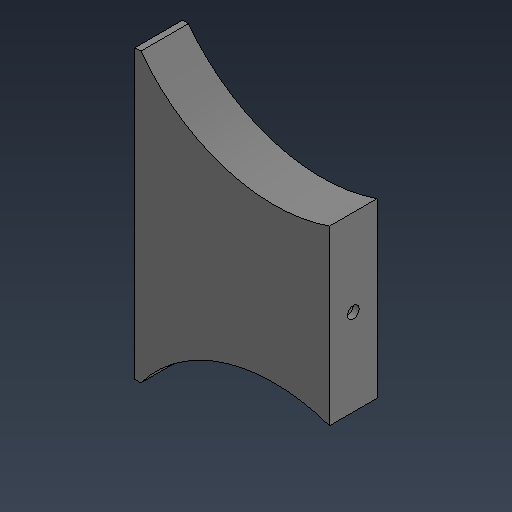
# Autodesk Inventor part: GearboxBearingHolderCover
Saved by Autodesk Inventor 2026.2 (Build 302298010, 298A)
## iProperties
Created: 2026-04-14
Part Number: GearboxBearingHolderCover
Material: Nylon 6/6
Document SubType Name: Modeling
Designer: szymo
Density: 1.13 g/cm^3
Appearance: Default(1)
Author: szymo
Autodesk Inventor part; units mm, degrees
ref_plane "YZ Plane" through (0, 0, 0) normal (1, 0, 0) x (0, 1, 0)
ref_plane "XZ Plane" through (0, 0, 0) normal (0, 1, 0) x (-1, 0, 0)
ref_plane "XY Plane" through (0, 0, 0) normal (0, 0, 1) x (1, 0, 0)
sketch "Sketch1" plane through (0, 0, 0) normal (0, 0, 1) x (1, 0, 0)
  line L0 (3.5, -23.1) -> (3, -23.1)
  line L1 (3, -23.1) -> (3, -47.2371)
  line L2 (3, -47.2371) -> (3.5, -47.2371)
  circle A0 centre (14.7, -14.7) radius 14
  circle A1 centre (14.7, -55.6371) radius 14
  circle A2 centre (14.7, -14.7) radius 14.7 construction
  line L3 (0, -14.7) -> (0, -55.6371) construction
  circle A3 centre (14.7, -55.6371) radius 14.7 construction
  circle A4 centre (12.35, -35.2722) radius 5
  line L4 (19.35, -27.9052) -> (19.35, -42.4319)
  circle A5 centre (14.7, -14.7) radius 14.7 projected
  circle A6 centre (14.7, -14.7) radius 14 projected
  circle A7 centre (14.7, -55.6371) radius 14.7 projected
  circle A8 centre (14.7, -55.6371) radius 14 projected
  circle A9 centre (12.35, -35.2722) radius 3.2 construction
  circle A10 centre (12.35, -35.2722) radius 4.8 construction
  point P0 (0, 0)
  dimension "d0" = 3
  dimension "d2" = 2
  dimension "d5" = 10
  dimension "d6" = 0.5
  dimension "d7" = 0.5
  dimension "d22" = 24.1371
  constraints: 10 end point, 5 coincident, 4 point on circle, 3 centre point, 3 vertical, 2 concentric, 2 horizontal alignment, 2 perpendicular, 1 horizontal, 6 other
  measures "d0" distance between parallel lines of L3 L1
  measures "d2" distance edge to line of A4 L4
  measures "d5" diameter of A4
  measures "d6" distance of L0.start L0.end
  measures "d7" distance of L1.end L2.end
  measures "d22" distance of L0.end L1.end
ref_plane "Work Plane1" through (5.5618, -42.0604, 3.6) normal (0, 0, 1) x (0.7075365, 0.7066768, 0)
extrude "Extrusion1" add sketch "Sketch1" along normal up to surface (3.6 mm away) contours A0 L4 A5 L1 L0 | A5 L4 A7 L1 | A7 L4 A1 L2 L1 picked at (4.6851, -25.0207) picked at (4.6851, -45.3164)
sketch "Sketch2" plane through (3, -47.2371, 3.6) normal (0, 0, 1) x (1, 0, 0)
  circle A0 centre (9.35, 11.9649) radius 5 projected
  line L0 (0, 0) -> (0, 24.1371) projected
  line L1 (0.5, 0) -> (0, 0) projected
  arc A1 (16.35, 4.8052) -> (0.5, 0) centre (11.7, -8.4) ccw projected
  line L2 (16.35, 19.3319) -> (16.35, 4.8052) projected
  arc A2 (0.5, 24.1371) -> (16.35, 19.3319) centre (11.7, 32.5371) ccw projected
  line L3 (0, 24.1371) -> (0.5, 24.1371) projected
  point P0 (-3, 47.2371)
extrude "Extrusion2" add sketch "Sketch2" along normal blind 0.4 contours A0 | L0 L3 A2 L2 A1 L1
sketch "Sketch3" plane through (3, -47.2371, 0) normal (-1, 0, 0) x (0, 0, 1)
  line L0 (0, 24.1371) -> (4, 24.1371) projected
  line L1 (0, 24.1371) -> (0, 0) projected
  line L2 (0, 0) -> (4, 0) projected
  line L3 (4, 24.1371) -> (4, 0) projected
  line L4 (4, 12.0685) -> (0, 12.0685) construction
  circle A0 centre (2, 17.0685) radius 2
  circle A1 centre (2, 7.0685) radius 2
  line L5 (0, 16.9649) -> (0, 6.9649) projected
  line L6 (0, 15.0685) -> (4, 15.0685) construction
  line L7 (0, 9.0685) -> (4, 9.0685) construction
  point P0 (0, 47.2371)
  dimension "d10" = 3
  dimension "d11" = 3
  constraints: 6 end point, 6 tangent, 4 point on line, 2 centre point, 2 midpoint, 2 perpendicular
  measures "d10" distance between parallel lines of L4 L7
  measures "d11" distance between parallel lines of L6 L4
hole "Hole1" at (3, -30.1685, 2) at (3, -40.1685, 2) direction (1, 0, 0) diameter 3 depth 5.5 counterbore diameter 3.5 counterbore depth 0.5
sketch "Sketch4" plane through (19.35, -42.4319, 0) normal (1, 0, 0) x (0, 0, -1)
  line L0 (0, 0) -> (-4, 0) projected
  line L1 (0, 0) -> (0, 14.5267) projected
  line L2 (0, 14.5267) -> (-4, 14.5267) projected
  line L3 (-4, 0) -> (-4, 14.5267) projected
  line L4 (0, 0) -> (-4, 14.5267)
  line L5 (0, 14.5267) -> (-4, 0)
  circle A0 centre (-2, 7.2633) radius 0.5
  point P0 (0, 42.4319)
  dimension "d19" = 1
  constraints: 4 end point, 1 centre point, 1 midpoint
  measures "d19" diameter of A0
extrude "Extrusion3" cut sketch "Sketch4" against normal blind 0.5 contours A0 L5 L4 | L4 L5 A0 | A0 L4 L5 | L5 L4 A0
equation "\"d7\" = d6"
equation "\"d10\" = d11"
body "Solid1"
